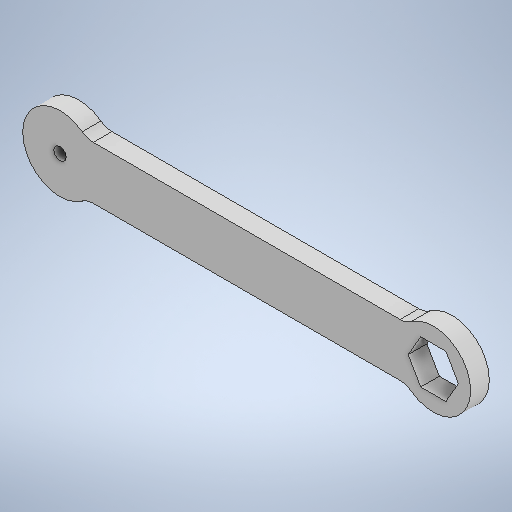
# Autodesk Inventor part: 2P.03.01.18.ZW.AileronCrank
Saved by Autodesk Inventor 2025.2 (Build 292293000, 293)
## iProperties
Created: 2025-01-14
Part Number: 2P.03.01.18.ZW.AileronCrank
Material: Generic
Document SubType Name: Modeling
Designer: Imist
Density: 1 g/cm^3
Appearance: Default
Author: Imist
Autodesk Inventor part; units mm, degrees
ref_plane "YZ Plane" through (0, 0, 0) normal (1, 0, 0) x (0, 1, 0)
ref_plane "XZ Plane" through (0, 0, 0) normal (0, 1, 0) x (-1, 0, 0)
ref_plane "XY Plane" through (0, 0, 0) normal (0, 0, 1) x (1, 0, 0)
sketch "Sketch1" plane through (0, 0, 0) normal (0, 0, 1) x (1, 0, 0)
  circle A0 centre (29.1378, 0) radius 3.5
  arc A1 (-30.8622, 6) -> (-30.8622, -6) centre (-30.8622, 0) ccw
  arc A2 (29.1378, -6) -> (29.1378, 6) centre (29.1378, 0) ccw
  arc A3 (-30.8622, -6) -> (-27.3004, -4.8284) centre (-30.8622, 0) ccw
  line L0 (-30.8622, 0) -> (-26.6195, -4.2426) construction
  line L1 (-30.8622, 0) -> (-30.8622, -6) construction
  arc A4 (-27.3004, 4.8284) -> (-30.8622, 6) centre (-30.8622, 0) ccw
  line L2 (-30.8622, 0) -> (-26.6195, 4.2426) construction
  line L3 (-30.8622, 0) -> (-30.8622, 6) construction
  arc A5 (29.1378, 6) -> (25.576, 4.8284) centre (29.1378, 0) ccw
  line L4 (29.1378, 0) -> (24.8952, 4.2426) construction
  line L5 (29.1378, 0) -> (29.1378, 6) construction
  arc A6 (25.576, -4.8284) -> (29.1378, -6) centre (29.1378, 0) ccw
  line L6 (29.1378, 0) -> (24.8952, -4.2426) construction
  line L7 (29.1378, 0) -> (29.1378, -6) construction
  line L8 (-25.5195, 4.2426) -> (23.7951, 4.2426)
  line L9 (-25.5195, -4.2426) -> (23.7951, -4.2426)
  arc A7 (-27.3004, 4.8284) -> (-25.5195, 4.2426) centre (-25.5195, 7.2426) ccw
  arc A8 (-25.5195, -4.2426) -> (-27.3004, -4.8284) centre (-25.5195, -7.2426) ccw
  arc A9 (23.7951, 4.2426) -> (25.576, 4.8284) centre (23.7951, 7.2426) ccw
  arc A10 (25.576, -4.8284) -> (23.7951, -4.2426) centre (23.7951, -7.2426) ccw
  line L10 (33.1793, 0) -> (31.1585, -3.5)
  line L11 (31.1585, -3.5) -> (27.1171, -3.5)
  line L12 (27.1171, -3.5) -> (25.0964, 0)
  line L13 (25.0964, 0) -> (27.1171, 3.5)
  line L14 (27.1171, 3.5) -> (31.1585, 3.5)
  line L15 (31.1585, 3.5) -> (33.1793, 0)
  circle A11 centre (-30.8622, 0) radius 1
  point P0 (0, 0)
  point P1 (24.8952, 4.2426)
  dimension "d1" = 7
  dimension "d2" = 60
  dimension "d3" = 6
  dimension "d4" = 6
  dimension "d5" = 45
  dimension "d6" = 45
  dimension "d7" = 45
  dimension "d8" = 45
  dimension "d9" = 3
  dimension "d17" = 2
  constraints: 32 end point, 24 point on circle, 12 centre point, 9 tangent, 8 coincident, 4 point on line, 3 equal radius, 2 horizontal alignment, 1 horizontal, 13 other
  measures "d1" diameter of A0
  measures "d2" distance of L1.end L7.end
  measures "d3" radius of A1
  measures "d4" radius of A2
  measures "d5" angle of L1 L0
  measures "d6" angle of L2 L3
  measures "d7" angle of L5 L4
  measures "d8" angle of L6 L7
  measures "d9" radius of A7
  measures "d17" diameter of A11
extrude "Extrusion2" add sketch "Sketch1" along normal blind 3
body "Solid2"
